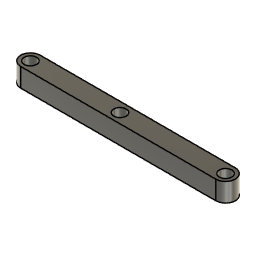
Moving_Stick3_ver4 v3 (Autodesk Fusion 360 design; units mm, degrees)
Autodesk Fusion 360 part; units mm, degrees
note: some values were not read from the file. Set by a fixed rule: which sketch regions a step uses.
sketch "스케치1" plane through (0, 0, 0) normal (0, 0, 1) x (1, 0, 0)
  line L0 (-25, -2.5) -> (25, -2.5)
  arc A0 (25, -2.5) -> (25, 2.5) centre (25, 0) ccw
  line L1 (25, 2.5) -> (-25, 2.5)
  arc A1 (-25, 2.5) -> (-25, -2.5) centre (-25, 0) ccw
  line L2 (-25, 0) -> (25, 0) construction
  circle A2 centre (25, 0) radius 1.6
  circle A3 centre (-25, 0) radius 1.6
  dimension "d1" = 5
  dimension "d2" = 3.2
  dimension "d3" = 3.2
  constraint tangent L0 A0
  constraint tangent A0 L1
  constraint parallel L0 L1
  constraint tangent L1 A1
  constraint tangent L0 A1
  constraint horizontal L2
  constraint concentric A0 A2
  constraint concentric A1 A3
  measures "d1" diameter of A0
  measures "d2" diameter of A2
  measures "d3" diameter of A3
extrude "돌출1" add sketch "스케치1" along normal blind 4.8
sketch "스케치2" plane through (0, 0, 4.8) normal (0, 0, 1) x (-1, 0, 0)
  circle A0 centre (-25, 0) radius 1.6
  circle A1 centre (25, 0) radius 1.6
  arc A2 (25, -2.5) -> (25, 2.5) centre (25, 0) ccw
  line L0 (25, 2.5) -> (-25, 2.5)
  arc A3 (-25, 2.5) -> (-25, -2.5) centre (-25, 0) ccw
  line L1 (-25, -2.5) -> (25, -2.5)
  line L2 (2.05, -15) -> (2.05, 10)
  circle A4 centre (2.05, 0) radius 1.6
  dimension "d7" = 3.2
  dimension "d10" = 27.05
  constraint vertical L2
  constraint coincident L2 A4.centre
  measures "d7" diameter of A4
  measures "d10" distance of A0.centre L2
extrude "돌출2" cut sketch "스케치2" against normal blind 5 contours L2 A4 | L2 A4
